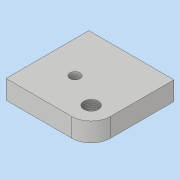
# Autodesk Inventor part: lw_6_part1
Saved by Autodesk Inventor 2022 (Build 260153000, 153)
## iProperties
Created: 2021-05-14
Part Number: lw_6_part1
Material: Типовые
Document SubType Name: Modeling
Designer: Kurbatova
Density: 1 g/cm^3
Appearance: По умолчанию
parametr_A_: 185,000 мм
parametr_B_: 180,000 мм
parametr_D_: 41,000 мм
parametr_E_: 35,000 мм
parametr_C_: 30,000 мм
parametr_F_: 20,000 мм
parametr_G_: 42,000 мм
parametr_H_: 100,000 мм
parametr_J_: 70,000 мм
Author: Kurbatova
Autodesk Inventor part; units mm, degrees
ref_plane "YZ Plane" through (0, 0, 0) normal (1, 0, 0) x (0, 1, 0)
ref_plane "XZ Plane" through (0, 0, 0) normal (0, 1, 0) x (-1, 0, 0)
ref_plane "XY Plane" through (0, 0, 0) normal (0, 0, 1) x (1, 0, 0)
sketch "Эскиз1" plane through (0, 0, 0) normal (0, 0, 1) x (1, 0, 0)
  line L0 (-88.1763, -30) -> (96.8237, -30)
  line L1 (-88.1763, -30) -> (-88.1763, 11)
  line L2 (96.8237, 11) -> (96.8237, -30)
  line L3 (-88.1763, 11) -> (96.8237, 11)
  point P0 (0, 0)
  point P1 (0, -30)
  dimension "parametr_A" = 185
  dimension "parametr_C" = 41
  constraints: 8 end point, 2 horizontal, 1 point on line, 1 vertical
  measures "parametr_A" distance of L0.start L0.end
  measures "parametr_C" distance of L1.end L0.start
extrude "Выдавливание2" add sketch "Эскиз1" along normal blind 180
fillet "Сопряжение1" radius 42 1 edges at (96.8237, -9.5, 180)
sketch "Эскиз5" plane through (-88.1763, -30, 0) normal (0, -1, 0) x (1, 0, 0)
  point P0 (70, 100)
hole "Отверстие5" at (-18.1763, -30, 100) direction (0, 1, 0) diameter 22 end through all
sketch "Эскиз7" plane through (-88.1763, 11, 0) normal (0, 1, 0) x (1, 0, 0)
  point P0 (143, -138)
hole "Отверстие7" at (54.8237, 11, 138) direction (0, -1, 0) diameter 31.67 depth 96 tip angle 120 thread size "M36x4" class "6H" standard "ISO Metric profile"
sketch "Эскиз2" plane through (-88.1763, -30, 0) normal (0, -1, 0) x (1, 0, 0)
  point P0 (114.3354, 27.5417)
sketch "Эскиз3" plane through (-88.1763, -30, 0) normal (0, -1, 0) x (1, 0, 0)
  point P0 (14.3354, 15.8973)
equation "\"parametr_A\" = parametr_A_"
equation "\"parametr_C\" = parametr_D_"
equation "\"paramert_B\" = parametr_B_"
equation "\"d21\" = parametr_G_"
equation "\"parametr_A_\" = 185"
equation "\"parametr_B_\" = 180"
equation "\"parametr_D_\" = 41"
equation "\"parametr_E_\" = 35"
equation "\"parametr_G_\" = 42"
